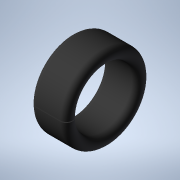
# Autodesk Inventor part: 8137184 ZBH-9-B
Saved by Autodesk Inventor 2021 (Build 250183000, 183)
## iProperties
Created: 2025-06-19
Part Number: 8137184 ZBH-9-B
Material: Generic
Catalog Web Link: www.cadenas.de
Description: ZBH-B-centring sleeve
Vendor: FESTO
Document SubType Name: Modeling
Designer: psAdmin
Manufacturer: FESTO
Mass: 2 g
Surface Area: 2.33331 cm^2
Volume: 0.11357 cm^3
Density: 1 g/cm^3
Appearance: PSOLRGB-175-175-175
Category: PARTsolutions
Company: FESTO
Title: 8137184 ZBH-9-B
Author: Cadenas PARTsolutions
Comments: centring sleeve
PSOL_IDENT_0: {$CADENAS_DATA/23d-libs/festo/parts/z/zbh/zbh_b.prj},169 {VTYP=3D},{NB=8137184 ZBH-9-B},{LINA=813718
PSOL_IDENT_1: 4 ZBH-9-B},{NN=ZBH-B},{DATE=02.05.2024 17:22:15},{GEOMDATE=28.07.2023 08:56:26},{VERSION=},{LINEID=8
PSOL_IDENT_2: 0},{WBVAR=},{WBNUMERIC=}  {NB=8137184 ZBH-9-B},{LINA=8137184 ZBH-9-B},{KT=DUMMY},{TNR=8137184},{TYP=
PSOL_IDENT_3: ZBH-9-B},{B1=3.900},{D1=9.000},{D2=6.400},{CNSMASSEXACT=0.002},{GTIN=4052568556983}
NB: 8137184 ZBH-9-B
NN: ZBH-B
NT: centring sleeve
NBSYN: $TNR. $TYP.
LINA: 8137184 ZBH-9-B
CATALOG: Festo
TNR: 8137184
TYP: ZBH-9-B
B1: 3.9
D1: 9
D2: 6.4
CNSMASSEXACT: 0.002
GTIN: 4052568556983
SUPPLIER: FESTO
ARTICLENO: 8137184 ZBH-9-B
BOMINFO: 8137184 ZBH-9-B
CREATOR: CADENAS GmbH
Autodesk Inventor part; units mm, degrees
sketch "Sketch_3" plane through (0, 0, 0) normal (0, 0, 1) x (1, 0, 0)
  line L0 (3.9, 0) -> (0, 0)
  arc A0 (0.65, 4.5) -> (0.65, 3.2) centre (0.65, 3.85) ccw
  line L1 (0.65, 3.2) -> (3.25, 3.2)
  arc A1 (3.25, 3.2) -> (3.25, 4.5) centre (3.25, 3.85) ccw
  line L2 (3.25, 4.5) -> (0.65, 4.5)
  constraints: 6 end point, 4 point on circle, 2 centre point
revolve "Revolution1" add sketch "Sketch_3" angle 360 about axis through (3.9, 0, 0) along (-1, 0, 0)
sketch "Sketch_4" plane through (0, 0, 0) normal (1, 0, 0) x (0, 1, 0)
  arc A0 (0.0903, 5.4993) -> (-0.0903, 5.4993) centre (0, 0) ccw
  line L0 (-0.0903, 5.4993) -> (0, 2.9136)
  line L1 (0, 2.9136) -> (0.0903, 5.4993)
  constraints: 4 end point, 2 point on circle, 1 centre point
extrude "Extrusion1" cut sketch "Sketch_4" along normal blind 3.9
ref_plane "ANBAU_XY" through (0, 0, 0) normal (1, 0, 0) x (0, 0, -1)
ref_plane "ANBAU_YZ" through (0, 0, 0) normal (0, 0, -1) x (0, 1, 0)
ref_plane "ANBAU_ZX" through (0, 0, 0) normal (0, 1, 0) x (1, 0, 0)
ref_plane "insert_XY" through (0, 0, 0) normal (1, 0, 0) x (0, 0, -1)
ref_plane "insert_YZ" through (0, 0, 0) normal (0, 0, -1) x (0, 1, 0)
ref_plane "insert_ZX" through (0, 0, 0) normal (0, 1, 0) x (1, 0, 0)
ref_plane "schraube_punkt_XY" through (3.9, 0, 0) normal (1, 0, 0) x (0, 0, -1)
ref_plane "schraube_punkt_YZ" through (3.9, 0, 0) normal (0, 0, -1) x (0, 1, 0)
ref_plane "schraube_punkt_ZX" through (3.9, 0, 0) normal (0, 1, 0) x (1, 0, 0)
body "Solid1"
